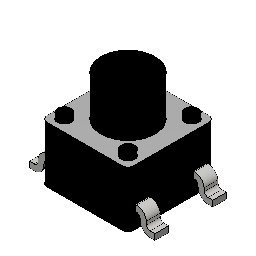
microswitch_4.5mm (Autodesk Fusion 360 design; units mm, degrees)
Autodesk Fusion 360 part; units mm, degrees
sketch "Sketch1" plane through (0, 0, 0) normal (0, 0, 1) x (1, 0, 0)
  line L0 (-1.95, 2.25) -> (1.95, 2.25)
  line L1 (2.25, 1.95) -> (2.25, -1.95)
  line L2 (1.95, -2.25) -> (-1.95, -2.25)
  line L3 (-2.25, -1.95) -> (-2.25, 1.95)
  arc A0 (-1.95, 2.25) -> (-2.25, 1.95) centre (-1.95, 1.95) ccw
  arc A1 (2.25, 1.95) -> (1.95, 2.25) centre (1.95, 1.95) ccw
  arc A2 (1.95, -2.25) -> (2.25, -1.95) centre (1.95, -1.95) ccw
  arc A3 (-2.25, -1.95) -> (-1.95, -2.25) centre (-1.95, -1.95) ccw
  line L4 (0, 2.25) -> (0, -2.25) construction
  point P0 (-2.25, 2.25)
  point P1 (2.25, 2.25)
  point P2 (-2.25, -2.25)
  dimension "d1" = 4.5
  dimension "d2" = 4.5
  dimension "d22" = 0.3
  constraint horizontal L0
  constraint vertical L1
  constraint horizontal L2
  constraint vertical L3
  constraint coincident P0 L0
  constraint coincident P0 L3
  constraint tangent L0 A0
  constraint tangent L3 A0
  constraint coincident P1 L0
  constraint coincident P1 L1
  constraint tangent L0 A1
  constraint tangent L1 A1
  constraint equal A0 A1
  constraint tangent L1 A2
  constraint tangent L2 A2
  constraint equal A0 A2
  constraint coincident P2 L2
  constraint coincident P2 L3
  constraint tangent L2 A3
  constraint tangent L3 A3
  constraint equal A0 A3
  constraint midpoint L0 L4.start
  constraint midpoint L2 L4.end
  constraint midpoint origin L4
  measures "d1" distance of P0 P2
  measures "d2" distance of P0 P1
  measures "d22" radius of A0
extrude "Extrude1" add sketch "Sketch1" along normal blind 2.9 makes body 1
sketch "Sketch3" plane through (0, 0, 2.9) normal (0, 0, 1) x (-1, 0, 0)
  line L0 (1.95, 2.25) -> (-1.95, 2.25)
  line L1 (-2.25, 1.95) -> (-2.25, -1.95)
  line L2 (-1.95, -2.25) -> (1.95, -2.25)
  line L3 (2.25, -1.95) -> (2.25, 1.95)
  circle A0 centre (0, 0) radius 1.4
  arc A1 (1.95, -2.25) -> (2.25, -1.95) centre (1.95, -1.95) ccw
  arc A2 (2.25, 1.95) -> (1.95, 2.25) centre (1.95, 1.95) ccw
  arc A3 (-1.95, 2.25) -> (-2.25, 1.95) centre (-1.95, 1.95) ccw
  arc A4 (-2.25, -1.95) -> (-1.95, -2.25) centre (-1.95, -1.95) ccw
  dimension "d5" = 2.8
  constraint coincident A0.centre origin
  measures "d5" diameter of A0
extrude "Extrude2" add sketch "Sketch3" along normal blind 5 from surface at -2.9 contours A0 bodies 1
sketch "Sketch4" plane through (0, 0, 0) normal (0, 1, 0) x (1, 0, 0)
  line L0 (-3.25, 0) -> (-3.25, -0.3)
  line L1 (-3.25, -0.3) -> (-3.0114, -0.3)
  line L2 (-2.8122, -0.4826) -> (-2.7981, -0.6436)
  line L3 (-2.3, -1.1) -> (-2.25, -1.1)
  line L4 (-3.25, 0) -> (-3.0114, 0)
  line L5 (-2.5133, -0.4564) -> (-2.4992, -0.6174)
  line L6 (-2.3, -0.8) -> (-2.25, -0.8)
  arc A0 (-2.4992, -0.6174) -> (-2.3, -0.8) centre (-2.3, -0.6) ccw
  arc A1 (-2.8122, -0.4826) -> (-3.0114, -0.3) centre (-3.0114, -0.5) ccw
  arc A2 (-2.7981, -0.6436) -> (-2.3, -1.1) centre (-2.3, -0.6) ccw
  arc A3 (-2.5133, -0.4564) -> (-3.0114, 0) centre (-3.0114, -0.5) ccw
  line L7 (-2.25, -1.1) -> (-2.25, -0.8)
  line L8 (-2.25, 0) -> (-2.25, -2.9)
  line L9 (-2.25, -2.9) -> (-2.25, 0) construction
  dimension "d9" = 3.25
  dimension "d10" = 0.3
  dimension "d11" = 1.1
  dimension "d13" = 0.3
  dimension "d14" = 85
  dimension "d18" = 0.5
  dimension "d23" = 0.05
  constraint vertical L0
  constraint horizontal L1
  constraint horizontal L3
  constraint horizontal L4
  constraint parallel L2 L5
  constraint horizontal L6
  constraint tangent L5 A0
  constraint tangent L6 A0
  constraint tangent L1 A1
  constraint tangent L2 A1
  constraint equal A0 A1
  constraint tangent L2 A2
  constraint tangent L3 A2
  constraint tangent L4 A3
  constraint tangent L5 A3
  constraint equal A2 A3
  constraint concentric A1 A3
  constraint collinear L7 L9
  constraint coincident L4 L8.start
  measures "d9" distance of origin L0
  measures "d10" distance of L0.start L0.end
  measures "d11" distance of L3 L4
  measures "d13" distance of L3 L6
  measures "d14" angle of L4 L5
  measures "d18" radius of A2
  measures "d23" distance of A0.centre L8
sketch "Sketch5" plane through (0, 0, 2.9) normal (0, 0, 1) x (-1, 0, 0)
  circle A0 centre (0, 0) radius 1.4
  arc A1 (1.95, -2.25) -> (2.25, -1.95) centre (1.95, -1.95) ccw
  line L0 (2.25, -1.95) -> (2.25, 1.95)
  arc A2 (2.25, 1.95) -> (1.95, 2.25) centre (1.95, 1.95) ccw
  line L1 (1.95, 2.25) -> (-1.95, 2.25)
  arc A3 (-1.95, 2.25) -> (-2.25, 1.95) centre (-1.95, 1.95) ccw
  line L2 (-2.25, 1.95) -> (-2.25, -1.95)
  arc A4 (-2.25, -1.95) -> (-1.95, -2.25) centre (-1.95, -1.95) ccw
  line L3 (-1.95, -2.25) -> (1.95, -2.25)
  circle A5 centre (1.65, -1.65) radius 0.35
  line L4 (0, 0) -> (0, -4.9) construction
  line L5 (0, 0) -> (6.7, 0) construction
  circle A6 centre (-1.65, -1.65) radius 0.35
  circle A7 centre (1.65, 1.65) radius 0.35
  circle A8 centre (-1.65, 1.65) radius 0.35
  dimension "d26" = 0.7
  dimension "d27" = 1.65
  dimension "d28" = 1.65
  constraint coincident A0.centre L4.start
  constraint vertical L4
  constraint perpendicular L4 L5
  constraint symmetric A5 L4 A6
  constraint symmetric A5 L5 A7
  constraint symmetric L5 A6 A8
  measures "d26" diameter of A5
  measures "d27" distance of A5.centre L5
  measures "d28" distance of A5.centre L4
extrude "Extrude4" add sketch "Sketch5" along normal blind 0.3 contours A5 | A6 | A7 | A8 bodies 1
extrude "Extrude3" add sketch "Sketch4" along normal mid plane 0.7 from surface at 1.5 separate body makes body 2
mirror "Mirror1" about plane through (0, 0, 0) normal (0, 1, 0) of bodies 2 makes body 3
mirror "Mirror2" about plane through (0, 0, 0) normal (1, 0, 0) of bodies 3 2 makes body 4 at (2.3247, 1.6167, 1.0994) makes body 5 at (2.3247, -1.6167, 1.0994)
equation "d9 = ( 6.5 / 2 ) * 1 mm"
